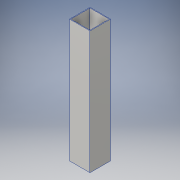
# Autodesk Inventor part: AlumPost-4x4x36-1_8
Saved by Autodesk Inventor 2016 SP1 (Build 200210100, 210)
## iProperties
Created: 2016-01-03
Part Number: AlumPost-4x4x36-1_8
Material: Aluminum 6061
Document SubType Name: Modeling
Designer: steele
Density: 2.7 g/cm^3
Appearance: Aluminum - Flat
Mass: 3086.09 g
Surface Area: 7224.99 cm^2
Volume: 1143 cm^3
Author: steele
Autodesk Inventor part; units mm, degrees
ref_plane "YZ Plane" through (0, 0, 0) normal (1, 0, 0) x (0, 1, 0)
ref_plane "XZ Plane" through (0, 0, 0) normal (0, 1, 0) x (-1, 0, 0)
ref_plane "XY Plane" through (0, 0, 0) normal (0, 0, 1) x (1, 0, 0)
sketch "Sketch1" plane through (0, 0, 0) normal (0, 1, 0) x (-1, 0, 0)
  line L0 (-50.8, 50.8) -> (-50.8, -50.8)
  line L1 (-50.8, -50.8) -> (50.8, -50.8)
  line L2 (50.8, -50.8) -> (50.8, 50.8)
  line L3 (50.8, 50.8) -> (-50.8, 50.8)
  line L4 (-50.8, 50.8) -> (50.8, -50.8) construction
  line L5 (-50.8, -50.8) -> (50.8, 50.8) construction
  line L6 (-47.625, 47.625) -> (-47.625, -47.625)
  line L7 (-47.625, -47.625) -> (47.625, -47.625)
  line L8 (47.625, -47.625) -> (47.625, 47.625)
  line L9 (47.625, 47.625) -> (-47.625, 47.625)
  line L10 (-47.625, 47.625) -> (47.625, -47.625) construction
  line L11 (-47.625, -47.625) -> (47.625, 47.625) construction
  point P0 (0, 0)
  dimension "d0" = 101.6
  dimension "d1" = 3.175
  constraints: 24 end point, 4 midpoint, 4 parallel, 4 perpendicular, 2 vertical
  measures "d0" distance of L0.start L0.end
  measures "d1" distance between parallel lines of L9 L3
extrude "Extrusion1" add sketch "Sketch1" along normal blind 609.6
body "Solid1"
